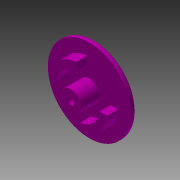
# Autodesk Inventor part: Kornylak Wheel Hub - Motor Side
Saved by Autodesk Inventor 2014 (Build 180170000, 170)
## iProperties
Created: 2014-02-14
Part Number: Kornylak Wheel Hub - Motor Side
Material: Generic
Document SubType Name: Modeling
Designer: Spooner
Density: 1 g/cm^3
Appearance: Magenta
Author: Spooner
Autodesk Inventor part; units mm, degrees
ref_plane "YZ Plane" through (0, 0, 0) normal (1, 0, 0) x (0, 1, 0)
ref_plane "XZ Plane" through (0, 0, 0) normal (0, 1, 0) x (-1, 0, 0)
ref_plane "XY Plane" through (0, 0, 0) normal (0, 0, 1) x (1, 0, 0)
sketch "Sketch1" plane through (0, 0, 0) normal (0, 0, 1) x (1, 0, 0)
  circle A0 centre (0, 0) radius 19.05
  dimension "d0" = 38.1
  constraints: 1 centre point, 1 coincident
  measures "d0" diameter of A0
extrude "Extrusion1" add sketch "Sketch1" along normal blind 2.54
sketch "Sketch2" plane through (0, 0, 2.54) normal (0, 0, 1) x (1, 0, 0)
  circle A0 centre (0, 0) radius 19.05 projected
  circle A1 centre (0, 0) radius 4.7371
  dimension "d3" = 9.4742
  constraints: 1 centre point, 1 coincident
  measures "d3" diameter of A1
extrude "Extrusion2" add sketch "Sketch2" along normal blind 8.509 contours A1
sketch "Sketch3" plane through (0, 0, 11.049) normal (0, 0, 1) x (1, 0, 0)
  circle A0 centre (0, 0) radius 4.7371 projected
  circle A1 centre (0, 0) radius 1.524
  dimension "d6" = 3.048
  constraints: 1 centre point, 1 coincident
  measures "d6" diameter of A1
extrude "Extrusion3" cut sketch "Sketch3" against normal through all contours A1
sketch "Sketch4" plane through (0, 0, 2.54) normal (0, 0, 1) x (1, 0, 0)
  circle A0 centre (0, 0) radius 4.7371 projected
  circle A1 centre (0, 0) radius 19.05 projected
  line L0 (-13.3346, 0.9271) -> (-9.8306, 0.9271)
  line L1 (-0.9271, 13.3346) -> (-0.9271, 9.8306)
  arc A2 (-0.9271, 13.3346) -> (-13.3346, 0.9271) centre (0, 0) ccw
  arc A3 (-0.9271, 9.8306) -> (-9.8306, 0.9271) centre (0, 0) ccw
  dimension "d9" = 0.9271
  dimension "d10" = 0.9271
  dimension "d11" = 9.8742
  dimension "d12" = 13.3667
  constraints: 4 end point, 4 point on circle, 2 centre point, 2 concentric, 1 horizontal, 1 perpendicular
  measures "d9" distance from line of A0.centre L0
  measures "d10" distance from line of A0.centre L1
  measures "d11" radius of A3
  measures "d12" radius of A2
extrude "Extrusion4" add sketch "Sketch4" along normal blind 5.08 contours A2 L1 A3 L0
pattern_circular "Circular Pattern1" count 2 over 360 about axis through (0, 0, 0) along (0, 0, 1) of "Extrusion4"
sketch "Sketch5" plane through (0, 0, 0) normal (0, 0, -1) x (-1, 0, 0)
  circle A0 centre (0, 0) radius 19.05 projected
  circle A1 centre (0, 0) radius 1.9304
  circle A2 centre (0, 0) radius 6.5532
  dimension "d18" = 3.8608
  dimension "d19" = 4.6228
  constraints: 2 centre point, 2 coincident
  measures "d18" diameter of A1
  measures "d19" radial gap between concentric circles of A1 A2
extrude "Extrusion5" add sketch "Sketch5" along normal blind 6.604 contours A2
sketch "Sketch6" plane through (0, 0, -6.604) normal (0, 0, -1) x (-1, 0, 0)
  circle A0 centre (0, 0) radius 1.9304 projected
  line L0 (-1.4756, 1.2446) -> (1.4756, 1.2446)
  arc A1 (1.4756, 1.2446) -> (-1.4756, 1.2446) centre (0, 0) ccw
  dimension "d22" = 3.175
  constraints: 4 point on circle, 2 end point, 1 centre point, 1 concentric, 1 horizontal
extrude "Extrusion6" add sketch "Sketch6" against normal up to surface (6.604 mm away) contours L0 A0 picked at (0.0798, 1.4682)
ref_plane "Work Plane1" through (0, 6.5532, 0) normal (0, -1, 0) x (1, 0, 0)
sketch "Sketch7" plane through (0, 6.5532, 0) normal (0, -1, 0) x (1, 0, 0)
  circle A0 centre (0, -3.302) radius 1.8415
  line L0 (-19.05, 0) -> (19.05, 0) projected
  line L1 (-6.5532, -6.604) -> (6.5532, -6.604) projected
  point P0 (0, 0)
  dimension "d25" = 3.683
  dimension "d26" = 3.302
  constraints: 1 centre point
  measures "d25" diameter of A0
  measures "d26" distance from line of L1 A0.centre
extrude "Extrusion7" cut sketch "Sketch7" along normal blind 6.35
fillet "Fillet1" radius 1.27 1 edges at (-19.05, 0, 0)
fillet "Fillet2" radius 1.27 1 edges at (6.5532, 0, 0)
equation "\"d10\" = d9"
body "Solid1"
